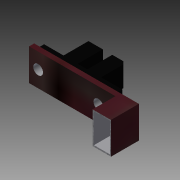
# Autodesk Inventor part: optical stop
Saved by Autodesk Inventor 2015 SP1 (Build 190203100, 203)
## iProperties
Created: 2015-02-07
Part Number: optical stop
Material: Generic
Document SubType Name: Modeling
Designer: Joseph
Density: 1 g/cm^3
Appearance: Default
Author: Joseph
Autodesk Inventor part; units mm, degrees
ref_plane "YZ Plane" through (0, 0, 0) normal (1, 0, 0) x (0, 1, 0)
ref_plane "XZ Plane" through (0, 0, 0) normal (0, 1, 0) x (-1, 0, 0)
ref_plane "XY Plane" through (0, 0, 0) normal (0, 0, 1) x (1, 0, 0)
sketch "Sketch1" plane through (0, 0, 0) normal (0, 0, 1) x (1, 0, 0)
  line L0 (-8.7842, -2.2796) -> (15.8158, -2.2796)
  line L1 (15.8158, -2.2796) -> (15.8158, 0.8304)
  line L2 (15.8158, 0.8304) -> (9.1958, 0.8304)
  line L3 (9.1958, 0.8304) -> (9.1958, 7.7401)
  line L4 (9.1958, 7.7401) -> (8.2439, 8.6704)
  line L5 (8.2439, 8.6704) -> (4.8058, 8.6704)
  line L6 (4.8058, 8.6704) -> (4.8058, 0.8304)
  line L7 (4.8058, 0.8304) -> (1.8458, 0.8304)
  line L8 (1.8458, 0.8304) -> (1.8458, 8.6704)
  line L9 (1.8458, 8.6704) -> (-2.6742, 8.6704)
  line L10 (-2.6742, 8.6704) -> (-2.6742, 0.8304)
  line L11 (-2.6742, 0.8304) -> (-8.7842, 0.8304)
  line L12 (-8.7842, 0.8304) -> (-8.7842, -2.2796)
  point P0 (0, 0)
  dimension "d0" = 24.6
  dimension "d1" = 3.11
  dimension "d2" = 4.39
  dimension "d3" = 2.96
  dimension "d4" = 4.52
  dimension "d5" = 6.62
  dimension "d6" = 7.84
  constraints: 26 end point, 7 perpendicular, 6 point on line, 1 horizontal, 1 parallel
  measures "d0" distance of L0.start L0.end
  measures "d1" distance of L0.end L1.end
  measures "d2" distance between parallel lines of L3 L6
  measures "d3" distance between parallel lines of L8 L6
  measures "d4" distance between parallel lines of L10 L8
  measures "d5" distance between parallel lines of L3 L1
  measures "d6" distance between parallel lines of L9 L11
extrude "Extrusion1" add sketch "Sketch1" along normal blind 6.43
sketch "Sketch2" plane through (9.1958, 0.8304, 0) normal (0, 1, 0) x (1, 0, 0)
  line L0 (6.62, 0) -> (0, 0) projected
  line L1 (6.62, -6.43) -> (0, -6.43) projected
  line L2 (6.62, 0) -> (6.62, -6.43) construction
  line L3 (6.62, -4.83) -> (-18.0124, -4.83) construction
  line L4 (-18.0124, -1.76) -> (6.62, -1.76) construction
  line L5 (-17.98, 0) -> (-17.98, -6.43) construction
  line L6 (-11.87, 0) -> (-17.98, 0) construction
  line L7 (-11.87, -6.43) -> (-17.98, -6.43) construction
  line L8 (-16.68, -6.43) -> (-16.68, 0) construction
  circle A0 centre (-15.145, -3.295) radius 1.535
  line L9 (5.32, 0) -> (5.32, -6.43) construction
  circle A1 centre (3.785, -3.295) radius 1.535
  point P0 (-9.1958, 0)
  dimension "d9" = 1.76
  dimension "d10" = 1.6
  dimension "d11" = 1.3
  dimension "d12" = 1.3
  constraints: 8 end point, 6 point on line, 6 tangent, 3 perpendicular, 2 centre point, 1 horizontal
  measures "d9" distance between parallel lines of L6 L4
  measures "d10" distance between parallel lines of L7 L3
  measures "d11" distance between parallel lines of L8 L5
  measures "d12" distance between parallel lines of L9 L2
extrude "Extrusion2" cut sketch "Sketch2" along normal up to surface (3.11 mm away) from surface at -3.11
sketch "Sketch3" plane through (-8.7842, -2.2796, 0) normal (0, -1, 0) x (1, 0, 0)
  circle A0 centre (2.835, 3.295) radius 1.535 projected
  circle A1 centre (21.765, 3.295) radius 1.535 projected
  line L0 (0, 0) -> (0, 6.43) projected
  line L1 (0, -1.785) -> (32.89, -1.785)
  line L2 (32.89, -1.785) -> (32.89, 8.215)
  line L3 (32.89, 8.215) -> (0, 8.215)
  line L4 (0, 8.215) -> (0, -1.785)
  line L5 (0, 3.215) -> (32.89, 3.215) construction
  point P0 (8.7842, 0)
  dimension "d15" = 32.89
  dimension "d16" = 10
  constraints: 10 end point, 3 midpoint, 2 parallel, 1 horizontal, 1 perpendicular
  measures "d15" distance of L3.end L2.end
  measures "d16" distance of L2.end L1.end
extrude "Extrusion3" add sketch "Sketch3" along normal blind 1.6
sketch "Sketch4" plane through (-8.7842, -3.8796, 0) normal (0, -1, 0) x (1, 0, 0)
  line L0 (0, -1.785) -> (32.89, -1.785) projected
  line L1 (32.89, 8.215) -> (27.11, 8.215)
  line L2 (27.11, 8.215) -> (27.11, -1.785)
  line L3 (27.11, -1.785) -> (32.89, -1.785)
  line L4 (32.89, -1.785) -> (32.89, 8.215)
  point P0 (8.7842, 0)
  dimension "d19" = 5.78
  constraints: 8 end point, 2 parallel, 1 horizontal, 1 perpendicular, 1 point on line
  measures "d19" distance of L3.end L2.end
extrude "Extrusion4" add sketch "Sketch4" along normal blind 7.17
sketch "Sketch5" plane through (-8.7842, -11.0496, 0) normal (0, -1, 0) x (1, 0, 0)
  line L0 (27.5471, -1.3186) -> (32.5822, -1.3186)
  line L1 (32.5822, -1.3186) -> (32.5822, 7.8489)
  line L2 (32.5822, 7.8489) -> (27.5471, 7.8489)
  line L3 (27.5471, 7.8489) -> (27.5471, -1.3186)
  point P0 (8.7842, 0)
  constraints: 8 end point, 2 parallel, 1 horizontal, 1 perpendicular
extrude "Extrusion5" cut sketch "Sketch5" against normal blind 7.33
body "Solid1"
